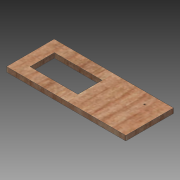
# Autodesk Inventor part: plaat1
Saved by Autodesk Inventor 2015 (Build 190159000, 159)
## iProperties
Created: 2016-01-31
Part Number: plaat1
Material: Generic
Document SubType Name: Modeling
Designer: david
Density: 1 g/cm^3
Appearance: Birch - Natural Polished
Author: david
Autodesk Inventor part; units mm, degrees
ref_plane "YZ Plane" through (0, 0, 0) normal (1, 0, 0) x (0, 1, 0)
ref_plane "XZ Plane" through (0, 0, 0) normal (0, 1, 0) x (-1, 0, 0)
ref_plane "XY Plane" through (0, 0, 0) normal (0, 0, 1) x (1, 0, 0)
sketch "Sketch1" plane through (0, 0, 0) normal (0, 0, 1) x (1, 0, 0)
  line L0 (-34.0226, 19.6334) -> (65.9774, 19.6334)
  line L1 (65.9774, 19.6334) -> (65.9774, -20.3666)
  line L2 (65.9774, -20.3666) -> (-34.0226, -20.3666)
  line L3 (-34.0226, -20.3666) -> (-34.0226, 19.6334)
  point P0 (0, 0)
  dimension "d0" = 100
  dimension "d1" = 40
  constraints: 8 end point, 2 parallel, 1 horizontal, 1 perpendicular
  measures "d0" distance of L1.end L2.end
  measures "d1" distance of L0.end L1.end
extrude "Extrusion1" add sketch "Sketch1" along normal blind 3.6
sketch "Sketch2" plane through (0, 0, 3.6) normal (0, 0, 1) x (1, 0, 0)
  line L0 (15.9774, -10.5166) -> (-24.0226, -10.5166)
  line L1 (-24.0226, -10.5166) -> (-24.0226, 9.7834)
  line L2 (-24.0226, 9.7834) -> (15.9774, 9.7834)
  line L3 (15.9774, 9.7834) -> (15.9774, -10.5166)
  line L4 (-34.0226, -20.3666) -> (65.9774, -20.3666) projected
  line L5 (65.9774, 19.6334) -> (-34.0226, 19.6334) projected
  line L6 (-34.0226, -20.3666) -> (-34.0226, 19.6334) projected
  point P0 (0, 0)
  dimension "d4" = 40
  dimension "d5" = 20.3
  dimension "d6" = 9.85
  dimension "d7" = 9.85
  dimension "d8" = 10
  constraints: 8 end point, 2 parallel, 1 horizontal, 1 perpendicular
  measures "d4" distance of L1.end L2.end
  measures "d5" distance of L0.end L1.end
  measures "d6" distance between parallel lines of L4 L0
  measures "d7" distance between parallel lines of L5 L2
  measures "d8" distance between parallel lines of L6 L1
extrude "Extrusion2" cut sketch "Sketch2" against normal blind 4
sketch "Sketch3" plane through (0, 0, 3.6) normal (0, 0, 1) x (1, 0, 0)
  line L0 (65.9774, -20.3666) -> (65.9774, 19.6334) projected
  circle A0 centre (65.9774, -0.3666) radius 20
  point P0 (0, 0)
  constraints: 1 midpoint, 1 vertical alignment, 2 other
extrude "Extrusion3" add sketch "Sketch3" against normal blind 3.6
sketch "Sketch4" plane through (0, 0, 3.6) normal (0, 0, 1) x (1, 0, 0)
  arc A0 (65.9774, -20.3666) -> (65.9774, 19.6334) centre (65.9774, -0.3666) ccw projected
  circle A1 centre (65.9774, -0.3666) radius 5.25
  point P0 (0, 0)
  dimension "d13" = 10.5
  constraints: 1 centre point, 1 coincident
  measures "d13" diameter of A1
extrude "Extrusion4" cut sketch "Sketch4" against normal blind 4
body "Solid1"
